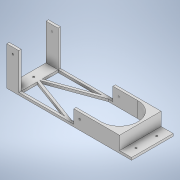
# Autodesk Inventor part: frame
Saved by Autodesk Inventor 2020 (Build 240168000, 168)
## iProperties
Created: 2020-02-29
Part Number: frame
Material: Типовые
Document SubType Name: Modeling
Designer: CSS38
Density: 1 g/cm^3
Appearance: По умолчанию
Author: CSS38
Autodesk Inventor part; units mm, degrees
ref_plane "YZ Plane" through (0, 0, 0) normal (1, 0, 0) x (0, 1, 0)
ref_plane "XZ Plane" through (0, 0, 0) normal (0, 1, 0) x (-1, 0, 0)
ref_plane "XY Plane" through (0, 0, 0) normal (0, 0, 1) x (1, 0, 0)
sketch "Эскиз1" plane through (0, 0, 0) normal (0, 1, 0) x (-1, 0, 0)
  line L0 (-51.75, 17.25) -> (51.75, 17.25)
  line L1 (51.75, 17.25) -> (51.75, -17.25)
  line L2 (51.75, -17.25) -> (-51.75, -17.25)
  line L3 (-51.75, -17.25) -> (-51.75, 17.25)
  line L4 (-51.75, 17.25) -> (51.75, -17.25) construction
  line L5 (51.75, 17.25) -> (-51.75, -17.25) construction
  line L6 (-41.75, -15.25) -> (0, -15.25)
  line L7 (41.75, -15.25) -> (41.75, -2.1292)
  line L8 (41.75, 15.25) -> (5.8292, 15.25)
  line L9 (-41.75, 15.25) -> (-41.75, -15.25)
  line L10 (0, -24.15) -> (0, 24.15) construction
  line L11 (0, -17.25) -> (0, -15.25) construction
  line L12 (0, 15.25) -> (0, 17.25) construction
  line L13 (0, -15.25) -> (41.75, 0)
  line L14 (41.75, 0) -> (0, 15.25)
  line L15 (5.8292, 15.25) -> (41.75, 2.1292)
  line L16 (41.75, -2.1292) -> (5.8292, -15.25)
  line L17 (41.75, -2.1292) -> (41.75, 2.1292) construction
  line L18 (41.75, 2.1292) -> (41.75, 15.25)
  line L19 (5.8292, -15.25) -> (41.75, -15.25)
  line L20 (0, -15.25) -> (5.8292, -15.25) construction
  line L21 (5.8292, 15.25) -> (0, 15.25) construction
  line L22 (0, 15.25) -> (-41.75, 15.25)
  line L23 (41.75, -2.1292) -> (41.0638, -0.2506) construction
  line L24 (41.75, 2.1292) -> (41.0638, 0.2506) construction
  point P0 (0, 0)
  point P1 (0, 0)
  dimension "d0" = 103.5
  dimension "d4" = 10
  dimension "d5" = 10
  dimension "d24" = 30.5
  dimension "d28" = 2
  constraints: 48 end point, 16 parallel, 16 perpendicular, 4 midpoint, 4 point on line, 3 equal length, 2 collinear, 1 coincident, 1 horizontal
  measures "d0" distance of L1.end L2.end
  measures "d4" distance between parallel lines of L7 L1
  measures "d5" distance between parallel lines of L9 L3
  measures "d24" distance of L9.start L6.start
  measures "d28" distance of L11.start L6.end
extrude "Выдавливание1" add sketch "Эскиз1" along normal blind 2
sketch "Эскиз2" plane through (0, 0, 0) normal (0, 1, 0) x (-1, 0, 0)
  line L0 (-41.75, -17.25) -> (-41.75, 17.25)
  line L1 (51.75, 17.25) -> (-51.75, 17.25) projected
  line L2 (-51.75, 17.25) -> (-51.75, -17.25) projected
  line L3 (0, -15.25) -> (-41.75, -15.25) construction
  line L4 (-39.75, -15.25) -> (-39.75, 15.25) construction
  line L5 (5.8292, 15.25) -> (41.75, 15.25) construction
  line L6 (-39.75, -15.25) -> (-24.5, -15.25) construction
  line L7 (-3.75, -15.25) -> (-3.75, -17.25)
  line L8 (-51.75, -17.25) -> (51.75, -17.25) projected
  line L9 (-3.75, -17.25) -> (-41.75, -17.25)
  line L10 (-41.75, 17.25) -> (-3.75, 17.25)
  line L11 (-3.75, 15.25) -> (-24.5, 15.25)
  line L12 (-3.75, 15.25) -> (-3.75, 17.25)
  arc A0 (-24.5, 15.25) -> (-24.5, -15.25) centre (-24.5, 0) ccw
  line L13 (-24.5, -15.25) -> (-3.75, -15.25)
  line L14 (-24.5, 15.25) -> (-39.75, 15.25) construction
  line L15 (-41.75, -15.25) -> (-41.75, 15.25) projected
  point P0 (0, 0)
  point P1 (41.75, -15.25)
  dimension "d13" = 2
  dimension "d14" = 36
  constraints: 20 end point, 7 point on line, 5 tangent, 4 collinear, 3 perpendicular, 3 vertical, 2 point on circle, 1 centre point
  measures "d13" distance between parallel lines of L0 L4
  measures "d14" distance of L4.start L7.start
extrude "Выдавливание2" add sketch "Эскиз2" along normal blind 13 contours L0 L1 L12 L11 A0 L13 L7 L8
sketch "Эскиз3" plane through (0, 2, 0) normal (0, 1, 0) x (1, 0, 0)
  line L0 (-41.75, 15.25) -> (-51.75, 15.25)
  line L1 (-51.75, 15.25) -> (-51.75, 17.25)
  line L2 (-51.75, 17.25) -> (-41.75, 17.25)
  line L3 (-41.75, 17.25) -> (-41.75, 15.25)
  line L4 (-51.75, 17.25) -> (-51.75, -17.25) construction
  line L5 (-51.75, -17.25) -> (-41.75, -17.25)
  line L6 (-41.75, -17.25) -> (-41.75, -15.25)
  line L7 (-41.75, -15.25) -> (-51.75, -15.25)
  line L8 (-51.75, -15.25) -> (-51.75, -17.25)
  point P0 (0, 0)
  point P1 (3.75, -15.25)
  constraints: 16 end point, 4 parallel, 2 coincident, 2 horizontal, 2 perpendicular
extrude "Выдавливание3" add sketch "Эскиз3" along normal blind 30
sketch "Эскиз5" plane through (0, 2, 0) normal (0, 1, 0) x (1, 0, 0)
  line L0 (51.75, 17.25) -> (51.75, -17.25) construction
  line L1 (51.75, -17.25) -> (41.75, -17.25) construction
  line L2 (41.75, 17.25) -> (41.75, -17.25) construction
  line L3 (3.75, 17.25) -> (41.75, 17.25) construction
  line L4 (3.75, 15.25) -> (3.75, 17.25) construction
  line L5 (3.75, 15.25) -> (0, 15.25) construction
  line L6 (0, 15.25) -> (-41.75, 0) construction
  line L7 (-41.75, 0) -> (0, -15.25) construction
  line L8 (0, -15.25) -> (3.75, -15.25) construction
  line L9 (3.75, -15.25) -> (24.5, -15.25) construction
  arc A0 (24.5, -15.25) -> (24.5, 15.25) centre (24.5, 0) ccw construction
  line L10 (24.5, 15.25) -> (3.75, 15.25) construction
  line L11 (41.75, 17.25) -> (51.75, 17.25) construction
  line L12 (41.75, -17.25) -> (3.75, -17.25) construction
  line L13 (3.75, -17.25) -> (3.75, -15.25) construction
  line L14 (-41.75, 17.25) -> (3.75, 17.25) construction
  line L15 (-41.75, 17.25) -> (-41.75, 15.25) construction
  line L16 (-5.8292, 15.25) -> (-41.75, 15.25) construction
  line L17 (-41.75, 2.1292) -> (-5.8292, 15.25) construction
  line L18 (-41.75, 15.25) -> (-41.75, 2.1292) construction
  line L19 (-41.75, 15.25) -> (-51.75, 15.25) construction
  line L20 (-51.75, 15.25) -> (-51.75, 17.25) construction
  line L21 (-51.75, 17.25) -> (-41.75, 17.25) construction
  line L22 (3.75, -17.25) -> (-41.75, -17.25) construction
  line L23 (-41.75, -15.25) -> (-41.75, -17.25) construction
  line L24 (-51.75, -15.25) -> (-41.75, -15.25) construction
  line L25 (-51.75, -17.25) -> (-51.75, -15.25) construction
  line L26 (-41.75, -17.25) -> (-51.75, -17.25) construction
  line L27 (-51.75, -15.25) -> (-51.75, 15.25) construction
  line L28 (-41.75, -15.25) -> (-5.8292, -15.25) construction
  line L29 (-5.8292, -15.25) -> (-41.75, -2.1292) construction
  line L30 (-41.75, -2.1292) -> (-41.75, -15.25) construction
  line L31 (-51.75, 17.25) -> (-41.75, -17.25) construction
  line L32 (-41.75, 17.25) -> (-51.75, -17.25) construction
  line L33 (51.75, 17.25) -> (-51.75, 17.25) construction
  line L34 (51.75, 17.25) -> (41.75, 0) construction
  line L35 (41.75, 17.25) -> (51.75, 0) construction
  line L36 (51.75, -17.25) -> (51.75, 17.25) construction
  line L37 (51.75, -17.25) -> (41.75, 0) construction
  line L38 (41.75, -17.25) -> (51.75, 0) construction
  circle A1 centre (-46.75, 0) radius 0.5
  circle A2 centre (46.75, 8.625) radius 0.5
  circle A3 centre (46.75, -8.625) radius 0.5
  point P0 (0, 0)
  dimension "d29" = 1
  constraints: 12 end point, 5 midpoint, 3 centre point, 2 equal radius, 2 parallel
  measures "d29" diameter of A1
hole "Отверстие1" at (-46.75, 2, 0) at (46.75, 2, 8.625) at (46.75, 2, -8.625) direction (0, -1, 0) diameter 1 end through all countersink diameter 1.5 countersink angle 90
sketch "Эскиз4" plane through (-51.75, 0, 17.25) normal (0, 0, 1) x (1, 0, 0)
  line L0 (10, 32) -> (0, 32) construction
  line L1 (0, 32) -> (10, 32) construction
  line L2 (10, 32) -> (10, 22) construction
  line L3 (10, 22) -> (0, 22) construction
  line L4 (0, 22) -> (0, 32) construction
  line L5 (103.5, 0) -> (0, 0) construction
  line L6 (0, 0) -> (0, 32) construction
  line L7 (10, 32) -> (10, 2) construction
  line L8 (10, 2) -> (55.5, 2) construction
  line L9 (55.5, 2) -> (55.5, 13) construction
  line L10 (55.5, 13) -> (93.5, 13) construction
  line L11 (93.5, 13) -> (93.5, 2) construction
  line L12 (93.5, 2) -> (103.5, 2) construction
  line L13 (103.5, 2) -> (103.5, 0) construction
  line L14 (10, 2) -> (10, 32) construction
  line L15 (0, 0) -> (0, 32) construction
  line L16 (10, 22) -> (0, 32) construction
  line L17 (10, 32) -> (0, 22) construction
  circle A0 centre (5, 27) radius 0.5
  line L18 (55.5, 13) -> (65.5, 13) construction
  line L19 (65.5, 13) -> (65.5, 3) construction
  line L20 (65.5, 3) -> (55.5, 3) construction
  line L21 (55.5, 3) -> (55.5, 13) construction
  line L22 (65.5, 13) -> (55.5, 3) construction
  line L23 (55.5, 2) -> (55.5, 13) construction
  line L24 (55.5, 13) -> (65.5, 3) construction
  circle A1 centre (60.5, 8) radius 0.5
  line L25 (0, 32) -> (10, 32) projected
  point P0 (51.75, 0)
  dimension "d19" = 1
  dimension "d20" = 10
  dimension "d21" = 1
  constraints: 24 end point, 5 perpendicular, 4 parallel, 2 centre point, 2 horizontal, 2 midpoint, 1 collinear
  measures "d19" diameter of A0
  measures "d20" distance of L19.end L20.end
  measures "d21" diameter of A1
hole "Отверстие2" at (-46.75, 27, 17.25) at (8.75, 8, 17.25) direction (0, 0, -1) diameter 1 depth 17.25 countersink diameter 1.5 countersink angle 90
mirror "Зеркальное отражение1" about plane through (0, 0, 0) normal (0, 0, 1) of "Отверстие2"
